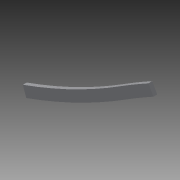
# Autodesk Inventor part: nd-g
Saved by Autodesk Inventor 2015 (Build 190159000, 159)
## iProperties
Created: 2014-07-02
Part Number: nd-g
Material: Generic
Document SubType Name: Modeling
Designer: peter
Density: 1 g/cm^3
Appearance: Default
Author: peter
Autodesk Inventor part; units mm, degrees
ref_plane "YZ Plane" through (0, 0, 0) normal (1, 0, 0) x (0, 1, 0)
ref_plane "XZ Plane" through (0, 0, 0) normal (0, 1, 0) x (-1, 0, 0)
ref_plane "XY Plane" through (0, 0, 0) normal (0, 0, 1) x (1, 0, 0)
sketch "Sketch1" plane through (0, 0, 0) normal (0, 0, 1) x (1, 0, 0)
  arc A0 (0, 47.9178) -> (483.371, 283.8081) centre (-821.207, 2343.8728) ccw
  line L0 (483.371, 283.8081) -> (483.3868, 283.8181)
  arc A1 (617.6605, 362.6596) -> (483.3868, 283.8181) centre (1784.548, -1778.4074) ccw
  line L1 (617.6605, 362.6596) -> (641.9707, 318.0541)
  arc A2 (641.9707, 318.0541) -> (510.5497, 240.89) centre (1784.548, -1778.4074) ccw
  arc A3 (17.1084, 0.0854) -> (510.5497, 240.89) centre (-821.2071, 2343.8737) ccw
  line L2 (17.1084, 0.0854) -> (0, 47.9178)
  constraints: 8 point on circle, 6 end point, 4 centre point
extrude "Extrusion1" add sketch "Sketch1" along normal blind 19.05
body "Solid1"
